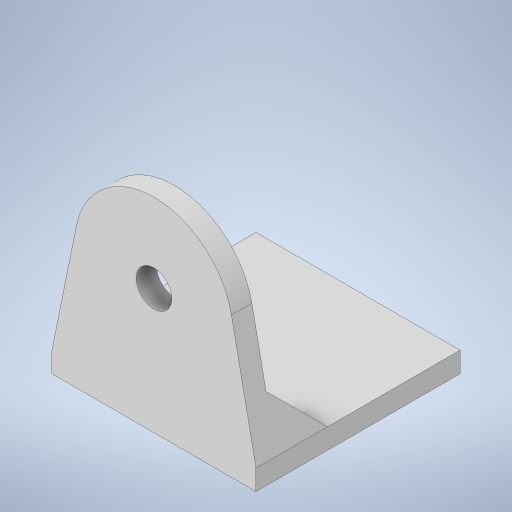
# Autodesk Inventor part: ChargingArm - FlatPlateBracket
Saved by Autodesk Inventor 2023 (Build 270158000, 158)
## iProperties
Created: 2023-04-05
Part Number: ChargingArm - FlatPlateBracket
Material: Generic
Document SubType Name: Modeling
Designer: Administrator
Density: 1 g/cm^3
Appearance: Default
Author: Administrator
Autodesk Inventor part; units mm, degrees
ref_plane "YZ Plane" through (0, 0, 0) normal (1, 0, 0) x (0, 1, 0)
ref_plane "XZ Plane" through (0, 0, 0) normal (0, 1, 0) x (-1, 0, 0)
ref_plane "XY Plane" through (0, 0, 0) normal (0, 0, 1) x (1, 0, 0)
sketch "Sketch1" plane through (0, 0, 0) normal (1, 0, 0) x (0, 1, 0)
  line L0 (0, 0) -> (20, 0)
  line L1 (20, 0) -> (20, -20)
  line L2 (20, -20) -> (0, -20)
  line L3 (0, -20) -> (0, 0)
  dimension "d0" = 20
  dimension "d1" = 20
  constraints: 8 end point, 2 parallel, 1 horizontal, 1 perpendicular
  measures "d0" distance of L1.end L2.end
  measures "d1" distance of L0.end L1.end
extrude "Extrusion1" add sketch "Sketch1" along normal blind 2
sketch "Sketch3" plane through (0, 20, 0) normal (0, 1, 0) x (1, 0, 0)
  circle A0 centre (12.25, 10) radius 7.75
  line L0 (2, 20) -> (2, 0) projected
  line L1 (2, 0) -> (13.7987, 2.4063)
  line L2 (2, 20) -> (13.7987, 17.5937)
  circle A1 centre (12.25, 10) radius 1.75
  point P0 (0, 0)
  point P1 (0, 20)
  dimension "d11" = 15.5
  dimension "d12" = 3.5
  constraints: 4 end point, 2 centre point, 2 point on circle, 2 tangent, 1 coincident, 1 equal length
  measures "d11" diameter of A0
  measures "d12" diameter of A1
extrude "Extrusion3" add sketch "Sketch3" against normal blind 2
chamfer "Chamfer3" distance 5 angle 45 1 edges at (2, 18, -10)
body "Solid1"
